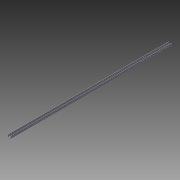
# Autodesk Inventor part: c hannel
Saved by Autodesk Inventor 2015 (Build 190159000, 159)
## iProperties
Created: 2015-01-10
Part Number: c hannel
Material: Generic
Document SubType Name: Modeling
Designer: bergjos18
Density: 1 g/cm^3
Appearance: Default
Author: bergjos18
Autodesk Inventor part; units mm, degrees
ref_plane "YZ Plane" through (0, 0, 0) normal (1, 0, 0) x (0, 1, 0)
ref_plane "XZ Plane" through (0, 0, 0) normal (0, 1, 0) x (-1, 0, 0)
ref_plane "XY Plane" through (0, 0, 0) normal (0, 0, 1) x (1, 0, 0)
sketch "Sketch1" plane through (0, 0, 0) normal (0, 0, 1) x (1, 0, 0)
  line L0 (0, 0) -> (0, 29.21)
  line L1 (0, 29.21) -> (3.81, 29.21)
  line L2 (3.81, 29.21) -> (3.81, 3.81)
  line L3 (3.81, 3.81) -> (29.21, 3.81)
  line L4 (29.21, 3.81) -> (29.21, 29.21)
  line L5 (29.21, 29.21) -> (33.02, 29.21)
  line L6 (33.02, 29.21) -> (33.02, 0)
  line L7 (33.02, 0) -> (0, 0)
  dimension "d0" = 29.21
  dimension "d1" = 3.81
  dimension "d2" = 25.4
  dimension "d3" = 25.4
  dimension "d4" = 3.81
  dimension "d48" = 3.81
  constraints: 16 end point, 5 perpendicular, 2 point on line, 1 parallel, 1 vertical
  measures "d0" distance of L0.start L0.end
  measures "d1" distance of L0.end L1.end
  measures "d2" distance of L1.end L2.end
  measures "d3" distance of L2.end L3.end
  measures "d4" distance of L4.end L5.end
  measures "d48" distance between parallel lines of L7 L3
extrude "Extrusion1" add sketch "Sketch1" along normal blind 1828.8
sketch "Sketch2" plane through (33.02, 29.21, 1828.8) normal (1, 0, 0) x (0, 0, -1)
  circle A0 centre (1816.1, -12.7) radius 3.175
  line L0 (1828.8, 0) -> (0, 0) projected
  line L1 (1828.8, 0) -> (1828.8, -29.21) projected
  circle A1 centre (1790.7, -12.7) radius 3.175
  circle A2 centre (1765.3, -12.7) radius 3.175
  circle A3 centre (1739.9, -12.7) radius 3.175
  circle A4 centre (1714.5, -12.7) radius 3.175
  circle A5 centre (1689.1, -12.7) radius 3.175
  circle A6 centre (1663.7, -12.7) radius 3.175
  circle A7 centre (1638.3, -12.7) radius 3.175
  circle A8 centre (1612.9, -12.7) radius 3.175
  circle A9 centre (1587.5, -12.7) radius 3.175
  circle A10 centre (1562.1, -12.7) radius 3.175
  circle A11 centre (1536.7, -12.7) radius 3.175
  circle A12 centre (1511.3, -12.7) radius 3.175
  circle A13 centre (1485.9, -12.7) radius 3.175
  circle A14 centre (1460.5, -12.7) radius 3.175
  circle A15 centre (1435.1, -12.7) radius 3.175
  circle A16 centre (1409.7, -12.7) radius 3.175
  circle A17 centre (1384.3, -12.7) radius 3.175
  circle A18 centre (1358.9, -12.7) radius 3.175
  circle A19 centre (1333.5, -12.7) radius 3.175
  circle A20 centre (1308.1, -12.7) radius 3.175
  circle A21 centre (1282.7, -12.7) radius 3.175
  circle A22 centre (1257.3, -12.7) radius 3.175
  circle A23 centre (1231.9, -12.7) radius 3.175
  circle A24 centre (1206.5, -12.7) radius 3.175
  circle A25 centre (1181.1, -12.7) radius 3.175
  circle A26 centre (1155.7, -12.7) radius 3.175
  circle A27 centre (1130.3, -12.7) radius 3.175
  circle A28 centre (1104.9, -12.7) radius 3.175
  circle A29 centre (1079.5, -12.7) radius 3.175
  circle A30 centre (1054.1, -12.7) radius 3.175
  circle A31 centre (1028.7, -12.7) radius 3.175
  circle A32 centre (1003.3, -12.7) radius 3.175
  circle A33 centre (977.9, -12.7) radius 3.175
  circle A34 centre (952.5, -12.7) radius 3.175
  circle A35 centre (927.1, -12.7) radius 3.175
  circle A36 centre (901.7, -12.7) radius 3.175
  circle A37 centre (876.3, -12.7) radius 3.175
  circle A38 centre (850.9, -12.7) radius 3.175
  circle A39 centre (825.5, -12.7) radius 3.175
  circle A40 centre (800.1, -12.7) radius 3.175
  circle A41 centre (774.7, -12.7) radius 3.175
  circle A42 centre (749.3, -12.7) radius 3.175
  circle A43 centre (723.9, -12.7) radius 3.175
  circle A44 centre (698.5, -12.7) radius 3.175
  circle A45 centre (673.1, -12.7) radius 3.175
  circle A46 centre (647.7, -12.7) radius 3.175
  circle A47 centre (622.3, -12.7) radius 3.175
  circle A48 centre (596.9, -12.7) radius 3.175
  circle A49 centre (571.5, -12.7) radius 3.175
  circle A50 centre (546.1, -12.7) radius 3.175
  circle A51 centre (520.7, -12.7) radius 3.175
  circle A52 centre (495.3, -12.7) radius 3.175
  circle A53 centre (469.9, -12.7) radius 3.175
  circle A54 centre (444.5, -12.7) radius 3.175
  circle A55 centre (419.1, -12.7) radius 3.175
  circle A56 centre (393.7, -12.7) radius 3.175
  circle A57 centre (368.3, -12.7) radius 3.175
  circle A58 centre (342.9, -12.7) radius 3.175
  circle A59 centre (317.5, -12.7) radius 3.175
  circle A60 centre (292.1, -12.7) radius 3.175
  circle A61 centre (266.7, -12.7) radius 3.175
  circle A62 centre (241.3, -12.7) radius 3.175
  circle A63 centre (215.9, -12.7) radius 3.175
  circle A64 centre (190.5, -12.7) radius 3.175
  circle A65 centre (165.1, -12.7) radius 3.175
  circle A66 centre (139.7, -12.7) radius 3.175
  circle A67 centre (114.3, -12.7) radius 3.175
  circle A68 centre (88.9, -12.7) radius 3.175
  circle A69 centre (63.5, -12.7) radius 3.175
  circle A70 centre (38.1, -12.7) radius 3.175
  circle A71 centre (12.7, -12.7) radius 3.175
  point P0 (1828.8, -22.225)
  dimension "d9" = 6.35
  dimension "d10" = 12.7
  dimension "d11" = 12.7
  dimension "d14" = 25.4
  dimension "d21" = 25.4
  constraints: 72 centre point, 2 horizontal, 142 other
  measures "d9" diameter of A0
  measures "d10" distance from line of L0 A0.centre
  measures "d11" distance from line of L1 A0.centre
  measures "d14" distance of A0.centre A1.centre
  measures "d21" distance of A70.centre A71.centre
hole "Hole1" at (33.02, 0, 0) at (33.02, 16.51, 12.7) at (33.02, 29.21, 0) at (33.02, 16.51, 165.1) at (33.02, 16.51, 139.7) at (33.02, 16.51, 114.3) at (33.02, 16.51, 88.9) at (33.02, 16.51, 63.5) at (33.02, 16.51, 38.1) at (33.02, 6.985, 0) at (33.02, 29.21, 1828.8) at (33.02, 16.51, 190.5) at (33.02, 16.51, 215.9) at (33.02, 16.51, 241.3) at (33.02, 16.51, 266.7) at (33.02, 16.51, 292.1) at (33.02, 16.51, 317.5) at (33.02, 16.51, 342.9) at (33.02, 16.51, 368.3) at (33.02, 16.51, 393.7) at (33.02, 16.51, 444.5) at (33.02, 16.51, 469.9) at (33.02, 16.51, 495.3) at (33.02, 16.51, 520.7) at (33.02, 16.51, 546.1) at (33.02, 16.51, 571.5) at (33.02, 16.51, 596.9) at (33.02, 16.51, 419.1) at (33.02, 16.51, 622.3) at (33.02, 16.51, 647.7) at (33.02, 16.51, 673.1) at (33.02, 16.51, 698.5) at (33.02, 16.51, 723.9) at (33.02, 16.51, 749.3) at (33.02, 16.51, 774.7) at (33.02, 16.51, 800.1) at (33.02, 16.51, 825.5) at (33.02, 16.51, 876.3) at (33.02, 16.51, 901.7) at (33.02, 16.51, 927.1) at (33.02, 16.51, 952.5) at (33.02, 16.51, 977.9) at (33.02, 16.51, 1003.3) at (33.02, 16.51, 850.9) at (33.02, 16.51, 1028.7) at (33.02, 16.51, 1054.1) at (33.02, 16.51, 1079.5) at (33.02, 16.51, 1104.9) at (33.02, 16.51, 1130.3) at (33.02, 16.51, 1155.7) direction (-1, 0, 0) diameter 6.35 end through all and at (33.02, 16.51, 1181.1) (33.02, 16.51, 1206.5) (33.02, 16.51, 1231.9) (33.02, 16.51, 1257.3) (33.02, 16.51, 1308.1) (33.02, 16.51, 1333.5) (33.02, 16.51, 1358.9) (33.02, 16.51, 1384.3) (33.02, 16.51, 1409.7) (33.02, 16.51, 1282.7) (33.02, 16.51, 1435.1) (33.02, 16.51, 1460.5) (33.02, 16.51, 1485.9) (33.02, 16.51, 1536.7) (33.02, 16.51, 1562.1) (33.02, 16.51, 1587.5) (33.02, 16.51, 1612.9) (33.02, 16.51, 1511.3) (33.02, 16.51, 1765.3) (33.02, 16.51, 1816.1) (33.02, 16.51, 1790.7) (33.02, 16.51, 1739.9) (33.02, 16.51, 1714.5) (33.02, 16.51, 1689.1) (33.02, 16.51, 1663.7) (33.02, 16.51, 1638.3)
sketch "Sketch3" plane through (33.02, 0, 3.175) normal (0, -1, 0) x (1, 0, 0)
  circle A0 centre (-16.51, 9.525) radius 3.175
  line L0 (0, 0) -> (0, 1825.625) projected
  line L1 (0, -3.175) -> (-3.81, -3.175) projected
  line L2 (0, 0) -> (0, -3.175) projected
  line L3 (-3.81, -3.175) -> (-3.81, 0) projected
  point P0 (-33.02, -3.175)
  dimension "d33" = 6.35
  dimension "d34" = 16.51
  dimension "d35" = 12.7
  dimension "d49" = 3.81
  constraints: 1 centre point
  measures "d33" diameter of A0
  measures "d34" distance from line of L0 A0.centre
  measures "d35" distance from line of L1 A0.centre
  measures "d49" distance between parallel lines of L2 L3
hole "Hole2" at (16.51, 0, 12.7) direction (0, 1, 0) diameter 6.35 end through all
pattern_linear "Rectangular Pattern1" count 72 spacing 25.4 along (0, 0, 1) of "Hole2"
fillet "Fillet3" radius 3.175 1 edges at (33.02, 0, 915.9875)
fillet "Fillet4" radius 3.175 1 edges at (0, 0, 915.9875)
body "Solid1"
